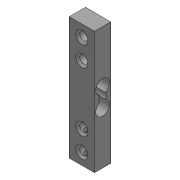
# Autodesk Inventor part: 20_020_LOAD_CELL_R2
Saved by Autodesk Inventor 2021.2 (Build 252289000, 289)
## iProperties
Created: 2018-02-01
Part Number: 20_020_LOAD_CELL_R2
Material: アルミニウム 6061
Document SubType Name: Modeling
Designer: y6tada
Density: 2.7 g/cm^3
Appearance: 滑らか - 標準の灰色
Mass: 5.03731 g
Surface Area: 18.822 cm^2
Volume: 1.86567 cm^3
Author: y6tada
Autodesk Inventor part; units mm, degrees
ref_plane "YZ Plane" through (0, 0, 0) normal (1, 0, 0) x (0, 1, 0)
ref_plane "XZ Plane" through (0, 0, 0) normal (0, 1, 0) x (-1, 0, 0)
ref_plane "XY Plane" through (0, 0, 0) normal (0, 0, 1) x (1, 0, 0)
sketch "スケッチ1" plane through (0, 0, 0) normal (1, 0, 0) x (0, 1, 0)
  line L0 (3, 22.53) -> (-3, 22.53)
  line L1 (-3, 22.53) -> (-3, -22.53)
  line L2 (-3, -22.53) -> (3, -22.53)
  line L3 (3, -22.53) -> (3, 22.53)
  line L4 (0, 22.53) -> (0, -22.53) construction
  line L5 (3, 0) -> (-3, 0) construction
  arc A0 (0.9953, 1.1222) -> (-0.9953, 1.1222) centre (0, 3.47) ccw
  arc A1 (-0.9953, -1.1222) -> (0.9953, -1.1222) centre (0, -3.47) ccw
  arc A2 (-0.9953, 1.1222) -> (-0.9953, -1.1222) centre (0, 0) ccw
  arc A3 (0.9953, -1.1222) -> (0.9953, 1.1222) centre (0, 0) ccw
  dimension "d0" = 6
  dimension "d1" = 45.06
  dimension "d3" = 5.1
  dimension "d4" = 12.04
  dimension "d5" = 1.5
  constraints: 12 end point, 8 point on circle, 5 midpoint, 4 centre point, 3 perpendicular, 3 symmetric about line, 2 coincident, 2 parallel, 1 concentric, 1 horizontal, 1 point on line, 3 other
  measures "d0" distance between parallel lines of L1 L3
  measures "d1" distance of L2.end L0.start
  measures "d3" diameter of A0
  measures "d5" radius of A3
extrude "押し出し1" add sketch "スケッチ1" along normal mid plane 9.3
sketch "スケッチ2" plane through (-4.65, 3, 22.53) normal (0, 1, 0) x (1, 0, 0)
  line L0 (4.65, 0) -> (4.65, 45.06) construction
  line L1 (9.3, 0) -> (0, 0) construction
  circle A0 centre (4.65, 4.23) radius 1.5
  circle A1 centre (4.65, 11.63) radius 1.5
  line L2 (9.3, 23.6522) -> (9.3, 21.4078) construction
  line L3 (9.3, 22.53) -> (-0.0401, 22.53) construction
  line L4 (9.3, 45.06) -> (0, 45.06) construction
  circle A2 centre (4.65, 40.83) radius 1.5
  circle A3 centre (4.65, 33.43) radius 1.5
  point P0 (4.65, 22.53)
  dimension "d8" = 21.8
  dimension "d9" = 7.4
  dimension "d10" = 3
  constraints: 6 end point, 5 midpoint, 4 centre point, 4 symmetric about line, 2 point on line, 1 equal radius, 1 horizontal, 1 vertical, 2 other
  measures "d8" diameter of A1.centre L3
  measures "d9" distance of A0.centre A1.centre
  measures "d10" diameter of A1
extrude "押し出し2" cut sketch "スケッチ2" against normal blind 6
chamfer "面取り1" distance 0.75 angle 45 8 edges at (-1.5, 3, 18.3) (-1.5, 3, 10.9) (-1.5, 3, -10.9) (-1.5, 3, -18.3) (-1.5, -3, 18.3) (-1.5, -3, 10.9) (-1.5, -3, -10.9) (-1.5, -3, -18.3)
sketch "スケッチ4" plane through (4.65, 3, -22.53) normal (0, 0, -1) x (-1, 0, 0)
  line L0 (4.65, -3) -> (4.65, -4) construction
  circle A0 centre (4.65, -4) radius 1
  line L1 (9.3, 0) -> (0, 0) construction
  dimension "d19" = 2
  dimension "d20" = 1
  dimension "d21" = 3
  constraints: 2 end point, 1 centre point, 1 coincident, 1 vertical
  measures "d19" diameter of A0
  measures "d20" distance of L0.start L0.end
  measures "d21" distance from line of L1 L0.start
extrude "押し出し4" cut sketch "スケッチ4" against normal blind 11.5
